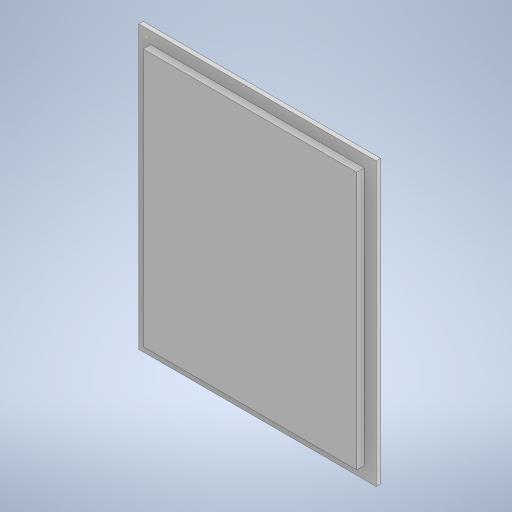
# Autodesk Inventor part: pokrywa
Saved by Autodesk Inventor 2023 (Build 270158000, 158)
## iProperties
Created: 2022-11-15
Part Number: pokrywa
Material: Generic
Document SubType Name: Modeling
Designer: Kamil
Density: 1 g/cm^3
Appearance: Default
Author: Kamil
Autodesk Inventor part; units mm, degrees
ref_plane "YZ Plane" through (0, 0, 0) normal (1, 0, 0) x (0, 1, 0)
ref_plane "XZ Plane" through (0, 0, 0) normal (0, 1, 0) x (-1, 0, 0)
ref_plane "XY Plane" through (0, 0, 0) normal (0, 0, 1) x (1, 0, 0)
sketch "Sketch1" plane through (0, 0, 0) normal (0, 0, 1) x (1, 0, 0)
  point P0 (0, 0)
sketch "Sketch2" plane through (0, 0, 0) normal (0, 0, 1) x (1, 0, 0)
  line L0 (0, 0) -> (149.8, 0)
  line L1 (149.8, 0) -> (149.8, -179.8)
  line L2 (149.8, -179.8) -> (0, -179.8)
  line L3 (0, -179.8) -> (0, 0)
  line L4 (0, -179.8) -> (160, -179.8)
  line L5 (160, -179.8) -> (160, 10.2)
  line L6 (0, 10.2) -> (0, -179.8)
  line L7 (0, 10.2) -> (160, 10.2)
  line L8 (-5.1, -184.9) -> (154.9, -184.9)
  line L9 (154.9, -184.9) -> (154.9, 5.1)
  line L10 (154.9, 5.1) -> (-5.1, 5.1)
  line L11 (-5.1, 5.1) -> (-5.1, -184.9)
  line L12 (146.8, -176.8) -> (3, -176.8)
  line L13 (3, -176.8) -> (3, -3)
  line L14 (3, -3) -> (146.8, -3)
  line L15 (146.8, -3) -> (146.8, -176.8)
  dimension "d21" = 5.1
  dimension "d22" = 190
  dimension "d23" = 160
  dimension "d28" = 8.1
  constraints: 32 end point, 7 parallel, 4 perpendicular, 3 horizontal, 6 other
  measures "d21" distance between parallel lines of L2 L8
  measures "d22" distance of L10.end L8.start
  measures "d23" distance of L8.start L8.end
  measures "d28" distance between parallel lines of L8 L12
extrude "Extrusion4" add sketch "Sketch2" against normal blind 3 contours L6 L10 L9 L4 L1 L0 | L0 L1 L2 L3 | L3 L2 L4 L9 L8 L11 L10 L6 | L12 L13 L14 L15
extrude "Extrusion6" add sketch "Sketch2" along normal blind 5 contours L12 L13 L14 L15
body "Solid2"
